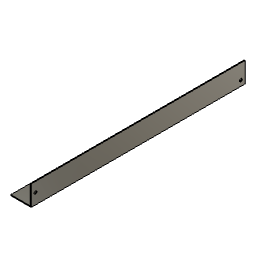
Bottom Angle 1.5 inch 400 mm Right v3 (Autodesk Fusion 360 design; units mm, degrees)
Autodesk Fusion 360 part; units mm, degrees
sketch "Sketch1" plane through (0, 0, 0) normal (0, 1, 0) x (1, 0, 0)
  line L0 (-38.1, 0) -> (0, 0)
  line L1 (0, 0) -> (0, -38.1)
  line L2 (-38.1, -1.5875) -> (-1.5875, -1.5875)
  line L3 (-1.5875, -1.5875) -> (-1.5875, -38.1)
  line L4 (-1.5875, -38.1) -> (0, -38.1)
  line L5 (-38.1, -1.5875) -> (-38.1, 0)
  dimension "d5" = 38.1
  dimension "d6" = 1.5875
  constraint horizontal L0
  constraint perpendicular L0 L1
  constraint coincident L0.end L1.start
  constraint equal L0 L1
  constraint perpendicular L1 L4
  constraint perpendicular L0 L5
  measures "d5" distance of L0.end L1.end
extrude "Extrude1" add sketch "Sketch1" along normal blind 400
sketch "Sketch3" plane through (-1.5875, 0, 0) normal (-1, 0, 0) x (0, -1, 0)
  line L0 (0, 1.5875) -> (0, 38.1)
  line L1 (0, 38.1) -> (-400, 38.1)
  line L2 (-400, 38.1) -> (-400, 1.5875)
  line L3 (-400, 1.5875) -> (0, 1.5875)
  circle A0 centre (-392, 10) radius 4.9317
  circle A1 centre (-8, 20) radius 5
  line L4 (0, 0) -> (-400, 0)
  dimension "d15" = 10
  dimension "d16" = 8
  dimension "d17" = 8
  dimension "d18" = 20
  measures "d15" distance of A0.centre L4
  measures "d16" distance of L2 A0.centre
  measures "d17" distance of L0 A1.centre
  measures "d18" distance of A1.centre L4
hole "Hole2" at (-1.5875, 8, 20) at (-1.5875, 392, 10) direction (1, 0, 0) diameter 5.5 depth 7 tip angle 118
sketch "Sketch4" plane through (0, 0, 1.5875) normal (0, 0, 1) x (-1, 0, 0)
  line L0 (38.1, 0) -> (1.5875, 0)
  line L1 (1.5875, 0) -> (1.5875, -400)
  line L2 (1.5875, -400) -> (38.1, -400)
  line L3 (38.1, -400) -> (38.1, 0)
  circle A0 centre (19.8375, -34.285) radius 6.9462
  circle A1 centre (19.8375, -365.715) radius 6.9462
  dimension "d22" = 34.285
  dimension "d23" = 34.285
  dimension "d24" = 18.25
  constraint vertical A0.centre A1.centre
  constraint equal A0 A1
  measures "d22" distance of L0 A0.centre
  measures "d23" distance of L2 A1.centre
  measures "d24" distance of L1 A1.centre
hole "Hole3" at (-19.8375, 34.285, 1.5875) at (-19.8375, 365.715, 1.5875) direction (0, 0, -1) diameter 5.5 depth 7 tip angle 118
